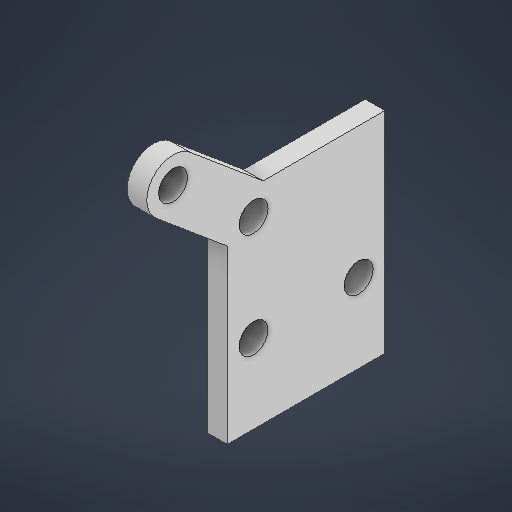
# Autodesk Inventor part: lifter arm mount
Saved by Autodesk Inventor 2026.1 (Build 301233020, 233B)
## iProperties
Created: 2025-11-05
Part Number: lifter arm mount
Material: Generic
Document SubType Name: Modeling
Designer: Asus
Density: 1 g/cm^3
Appearance: Default
Author: Asus
Autodesk Inventor part; units mm, degrees
ref_plane "YZ Plane" through (0, 0, 0) normal (1, 0, 0) x (0, 1, 0)
ref_plane "XZ Plane" through (0, 0, 0) normal (0, 1, 0) x (-1, 0, 0)
ref_plane "XY Plane" through (0, 0, 0) normal (0, 0, 1) x (1, 0, 0)
sketch "Sketch1" plane through (0, 0, 0) normal (1, 0, 0) x (0, 1, 0)
  line L0 (32, -24) -> (0, -24)
  line L1 (0, -24) -> (0, 0)
  circle A0 centre (12, -4) radius 2.2
  circle A1 centre (12, -20) radius 2.2
  circle A2 centre (28, -4) radius 2.2
  line L2 (32, -5.4559) -> (41.3488, 5.6856)
  line L3 (35.2204, 10.8279) -> (26.1348, 0)
  arc A3 (41.3488, 5.6856) -> (35.2204, 10.8279) centre (38.2846, 8.2567) ccw
  line L4 (28, -4) -> (48, -4) construction
  line L5 (32, -5.4559) -> (32, -24)
  line L6 (0, 0) -> (26.1348, 0)
  circle A4 centre (38.2846, 8.2567) radius 2.2
  point P0 (34.4279, 3.6604)
  dimension "d1" = 32
  dimension "d2" = 4.4
  dimension "d3" = 12
  dimension "d5" = 4.4
  dimension "d6" = 4
  dimension "d7" = 4.4
  dimension "d10" = 16
  dimension "d12" = 8
  dimension "d13" = 4.4
  constraints: 14 end point, 5 centre point, 3 parallel, 2 horizontal, 2 point on circle, 2 tangent, 1 coincident, 1 perpendicular, 1 other
  measures "d1" distance of L0.start L0.end
  measures "d2" diameter of A0
  measures "d3" distance from line of L1 A0.centre
  measures "d5" diameter of A1
  measures "d6" distance from line of L0 A1.centre
  measures "d7" diameter of A2
  measures "d10" distance of L4.start A3.centre
  measures "d12" diameter of A3
  measures "d13" diameter of A4
extrude "Extrusion1" add sketch "Sketch1" along normal blind 3
body "Solid1"
